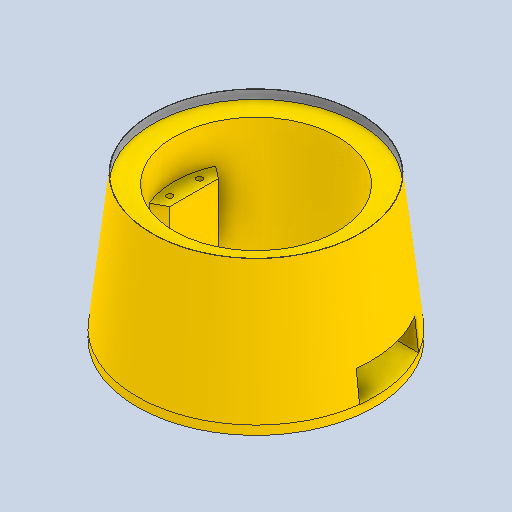
# Autodesk Inventor part: Base
Saved by Autodesk Inventor 2024 (Build 280153000, 153)
## iProperties
Created: 2024-04-28
Part Number: Base
Material: Generic
Document SubType Name: Modeling
Designer: samue
Density: 1 g/cm^3
Appearance: Default
Author: samue
Autodesk Inventor part; units mm, degrees
ref_plane "YZ Plane" through (0, 0, 0) normal (1, 0, 0) x (0, 1, 0)
ref_plane "XZ Plane" through (0, 0, 0) normal (0, 1, 0) x (-1, 0, 0)
ref_plane "XY Plane" through (0, 0, 0) normal (0, 0, 1) x (1, 0, 0)
sketch "Sketch1" plane through (0, 0, 0) normal (0, 1, 0) x (-1, 0, 0)
  circle A0 centre (0, 0) radius 40
  dimension "d0" = 80
  constraints: 1 centre point, 1 coincident
  measures "d0" diameter of A0
extrude "Extrusion1" add sketch "Sketch1" along normal blind 3
ref_plane "Work Plane1" through (0, 48, 0) normal (0, 1, 0) x (1, 0, 0)
sketch "Sketch2" plane through (0, 48, 0) normal (0, 1, 0) x (1, 0, 0)
  circle A0 centre (0, 0) radius 35
  dimension "d4" = 70
  constraints: 1 centre point, 1 coincident
  measures "d4" diameter of A0
loft "Loft1" add profiles "Sketch2" section 1 edges at (40, 3, 0)
sketch "Sketch3" plane through (0, 48, 0) normal (0, 1, 0) x (1, 0, 0)
  circle A0 centre (0, 0) radius 27.5
  dimension "d9" = 55
  constraints: 1 centre point, 1 coincident
  measures "d9" diameter of A0
extrude "Extrusion2" cut sketch "Sketch3" against normal blind 45
sketch "Sketch4" plane through (0, 3, 0) normal (0, 1, 0) x (1, 0, 0)
  line L0 (-24, 5) -> (24, 5)
  line L1 (24, 5) -> (24, -5)
  line L2 (24, -5) -> (-24, -5)
  line L3 (-24, -5) -> (-24, 5)
  line L4 (-24, 5) -> (24, -5) construction
  line L5 (24, 5) -> (-24, -5) construction
  circle A0 centre (-24, 5) radius 3
  circle A1 centre (-24, -5) radius 3
  circle A2 centre (24, 5) radius 3
  circle A3 centre (24, -5) radius 3
  point P0 (0, 0)
  dimension "d12" = 48
  dimension "d13" = 10
  dimension "d14" = 6
  dimension "d15" = 6
  dimension "d16" = 6
  dimension "d17" = 6
  constraints: 12 end point, 4 centre point, 4 coincident, 2 midpoint, 2 parallel, 1 horizontal, 1 perpendicular
  measures "d12" distance of L1.end L2.end
  measures "d13" distance of L0.end L1.end
  measures "d14" diameter of A0
  measures "d15" diameter of A1
  measures "d16" diameter of A2
  measures "d17" diameter of A3
extrude "Extrusion3" add sketch "Sketch4" along normal blind 29 contours L3 A0 L0 | L0 A0 L3 | A2 L1 L0 | L0 L1 A2 | A1 L2 L3 | L3 L2 A1 | A3 L2 L1 | L1 L2 A3
sketch "Sketch5" plane through (0, 48, 0) normal (0, 1, 0) x (1, 0, 0)
  circle A0 centre (0, 0) radius 34.8785
  constraints: 1 centre point, 1 coincident
extrude "Extrusion4" cut sketch "Sketch5" against normal blind 3
sketch "Sketch6" plane through (0, 32, 0) normal (0, 1, 0) x (1, 0, 0)
  arc A0 (-26.9855, 5.2946) -> (-26.8548, 5.9221) centre (-24, 5) ccw projected
  arc A1 (-26.9855, -5.2946) -> (-26.8548, -5.9221) centre (0, 0) ccw projected
  arc A2 (-26.8548, -5.9221) -> (-26.9855, -5.2946) centre (-24, -5) ccw projected
  arc A3 (26.9855, 5.2946) -> (26.8548, 5.9221) centre (0, 0) ccw projected
  arc A4 (26.8548, 5.9221) -> (26.9855, 5.2946) centre (24, 5) ccw projected
  arc A5 (26.8548, -5.9221) -> (26.9855, -5.2946) centre (0, 0) ccw projected
  arc A6 (26.9855, -5.2946) -> (26.8548, -5.9221) centre (24, -5) ccw projected
  circle A7 centre (-24, 5) radius 1
  circle A8 centre (24, 5) radius 1
  circle A9 centre (-24, -5) radius 1
  circle A10 centre (24, -5) radius 1
  dimension "d22" = 2
  dimension "d23" = 2
  dimension "d24" = 2
  dimension "d25" = 2
  constraints: 4 centre point, 4 coincident
  measures "d22" diameter of A7
  measures "d23" diameter of A8
  measures "d24" diameter of A9
  measures "d25" diameter of A10
sketch "Sketch7" plane through (0, 3, 0) normal (0, 1, 0) x (1, 0, 0)
  arc A0 (26.8548, 5.9221) -> (-26.8548, 5.9221) centre (0, 0) ccw projected
  arc A1 (-26.8548, -5.9221) -> (26.8548, -5.9221) centre (0, 0) ccw projected
  arc A2 (-25.014, 11.4257) -> (-25.3704, -10.611) centre (0, 0) ccw
  line L0 (-25.014, 11.4257) -> (-20.9048, 8.2442)
  line L1 (-20.9048, 8.2442) -> (-20.9088, -8.1021)
  line L2 (-20.9088, -8.1021) -> (-25.3704, -10.611)
  point P0 (-26.8548, 5.9221)
  point P1 (-26.8548, -5.9221)
  constraints: 6 end point, 4 point on circle, 1 centre point
extrude "Extrusion6" add sketch "Sketch7" along normal blind 29
mirror "Mirror1" about plane through (0, 0, 0) normal (1, 0, 0) of "Extrusion6"
extrude "Extrusion7" cut sketch "Sketch6" against normal blind 14 contours A7 | A8 | A9 | A10
sketch "Sketch8" plane through (20.9088, 3, 8.1021) normal (-1, 0, 0.0002409) x (0.0002409, 0, 1)
  line L0 (0, 0) -> (-16.3463, 0) projected
  line L1 (-28.2337, 0) -> (-3.2337, 0)
  line L2 (-3.2337, 0) -> (-3.2337, 10)
  line L3 (-3.2337, 10) -> (-28.2337, 10)
  line L4 (-28.2337, 10) -> (-28.2337, 0)
  point P0 (-8.1072, -3)
  point P1 (-16.3463, 0)
  dimension "d33" = 25
  dimension "d34" = 10
  constraints: 8 end point, 2 parallel, 1 horizontal, 1 perpendicular, 1 point on line
  measures "d33" distance of L3.end L2.end
  measures "d34" distance of L2.end L1.end
extrude "Extrusion8" cut sketch "Sketch8" against normal blind 20
sketch "Sketch9" plane through (20.9088, 3, 8.1021) normal (1, 0, -0.0002409) x (-0.0002409, 0, -1)
  line L0 (28.2337, 10) -> (28.2337, 0) projected
  line L1 (28.2337, 10) -> (25.9721, 10)
  line L2 (25.9721, 10) -> (25.9721, 0)
  line L3 (25.9721, 0) -> (28.2337, 0)
  line L4 (28.2337, 0) -> (28.2337, 10)
  point P0 (8.1072, -3)
  constraints: 8 end point, 2 parallel, 1 horizontal, 1 perpendicular
extrude "Extrusion9" cut sketch "Sketch9" against normal blind 20
body "Solid1"
